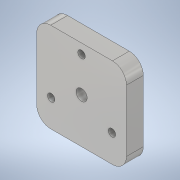
# Autodesk Inventor part: MiddleStandOff
Saved by Autodesk Inventor 2021 (Build 250183000, 183)
## iProperties
Created: 2020-04-08
Part Number: MiddleStandOff
Material: Generic
Document SubType Name: Modeling
Designer: lgnds
Density: 1 g/cm^3
Appearance: Default
Author: lgnds
Autodesk Inventor part; units mm, degrees
ref_plane "YZ Plane" through (0, 0, 0) normal (1, 0, 0) x (0, 1, 0)
ref_plane "XZ Plane" through (0, 0, 0) normal (0, 1, 0) x (-1, 0, 0)
ref_plane "XY Plane" through (0, 0, 0) normal (0, 0, 1) x (1, 0, 0)
sketch "Sketch1" plane through (0, 0, 0) normal (0, 0, 1) x (1, 0, 0)
  circle A0 centre (0, 0) radius 16 construction
  line L0 (-16, -16) -> (16, -16)
  line L1 (16, -16) -> (16, 16)
  line L2 (16, 16) -> (-16, 16)
  line L3 (-16, 16) -> (-16, -16)
  line L4 (-16, -16) -> (16, 16) construction
  line L5 (16, -16) -> (-16, 16) construction
  dimension "d0" = 32
  constraints: 12 end point, 2 midpoint, 2 parallel, 2 tangent, 1 centre point, 1 coincident, 1 horizontal, 1 perpendicular
  measures "d0" diameter of A0
extrude "Extrusion1" add sketch "Sketch1" along normal blind 6
sketch "Sketch2" plane through (0, 0, 6) normal (0, 0, 1) x (1, 0, 0)
  circle A0 centre (0, 0) radius 2
  dimension "d3" = 4
  constraints: 1 centre point, 1 coincident
  measures "d3" diameter of A0
extrude "Extrusion2" cut sketch "Sketch2" against normal up to surface (6 mm away)
fillet "Fillet1" radius 5 4 edges at (16, 16, 3) (16, -16, 3) (-16, -16, 3) (-16, 16, 3)
sketch "Sketch3" plane through (0, 0, 6) normal (0, 0, 1) x (1, 0, 0)
  circle A0 centre (0, 0) radius 2 construction
  circle A1 centre (0, 0) radius 12.5 construction
  line L0 (0, -22.4) -> (0, 22.4) construction
  line L1 (-22.4, 0) -> (22.4, 0) construction
  circle A2 centre (0, 12.5) radius 1.325
  circle A3 centre (10.8253, -6.25) radius 1.325
  circle A4 centre (-10.8253, -6.25) radius 1.325
  line L2 (0, 0) -> (22.5547, -13.0219) construction
  line L3 (0, 0) -> (-20.3118, -11.727) construction
  dimension "d7" = 25
  dimension "d8" = 2.65
  dimension "d9" = 2.65
  dimension "d10" = 2.65
  dimension "d11" = 30
  dimension "d12" = 30
  constraints: 4 centre point, 4 end point, 3 point on circle, 3 point on line, 1 coincident
  measures "d7" diameter of A1
  measures "d8" diameter of A2
  measures "d9" diameter of A3
  measures "d10" diameter of A4
  measures "d11" angle of L1 L3
  measures "d12" angle of L1 L2
extrude "Extrusion3" cut sketch "Sketch3" against normal through all
equation "\"d9\" = d8"
equation "\"d10\" = d8"
body "Solid1"
